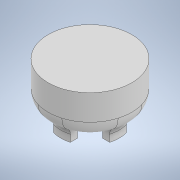
# Autodesk Inventor part: lower joint
Saved by Autodesk Inventor 2022 (Build 260153000, 153)
## iProperties
Created: 2022-03-14
Part Number: lower joint
Material: Generic
Document SubType Name: Modeling
Designer: RNG3nius
Density: 1 g/cm^3
Appearance: Default
Author: RNG3nius
Autodesk Inventor part; units mm, degrees
ref_plane "YZ Plane" through (0, 0, 0) normal (1, 0, 0) x (0, 1, 0)
ref_plane "XZ Plane" through (0, 0, 0) normal (0, 1, 0) x (-1, 0, 0)
ref_plane "XY Plane" through (0, 0, 0) normal (0, 0, 1) x (1, 0, 0)
sketch "Sketch1" plane through (0, 0, 0) normal (0, 1, 0) x (-1, 0, 0)
  circle A0 centre (0, 0) radius 5
  dimension "d0" = 10
  constraints: 1 centre point, 1 coincident
  measures "d0" diameter of A0
extrude "Extrusion1" add sketch "Sketch1" along normal blind 5
sketch "Sketch2" plane through (0, 0, 0) normal (0, -1, 0) x (1, 0, 0)
  circle A0 centre (0, 0) radius 3.5
  line L0 (1, -2.5) -> (-1, -2.5)
  line L1 (-1, -2.5) -> (-1, -4.5)
  line L2 (-1, -4.5) -> (1, -4.5)
  line L3 (1, -4.5) -> (1, -2.5)
  line L4 (1, -2.5) -> (-1, -4.5) construction
  line L5 (-1, -2.5) -> (1, -4.5) construction
  line L6 (4.5, 1) -> (2.5, 1)
  line L7 (2.5, 1) -> (2.5, -1)
  line L8 (2.5, -1) -> (4.5, -1)
  line L9 (4.5, -1) -> (4.5, 1)
  line L10 (4.5, 1) -> (2.5, -1) construction
  line L11 (2.5, 1) -> (4.5, -1) construction
  line L12 (1, 4.5) -> (-1, 4.5)
  line L13 (-1, 4.5) -> (-1, 2.5)
  line L14 (-1, 2.5) -> (1, 2.5)
  line L15 (1, 2.5) -> (1, 4.5)
  line L16 (1, 4.5) -> (-1, 2.5) construction
  line L17 (-1, 4.5) -> (1, 2.5) construction
  line L18 (-4.5, 1) -> (-2.5, 1)
  line L19 (-2.5, 1) -> (-2.5, -1)
  line L20 (-2.5, -1) -> (-4.5, -1)
  line L21 (-4.5, -1) -> (-4.5, 1)
  line L22 (-4.5, 1) -> (-2.5, -1) construction
  line L23 (-2.5, 1) -> (-4.5, -1) construction
  point P0 (0, -3.5)
  point P1 (3.5, 0)
  point P2 (0, 3.5)
  point P3 (-3.5, 0)
  point P4 (-3.3541, 1)
  point P5 (-3.3541, -1)
  point P6 (-1, -3.3541)
  point P7 (1, -3.3541)
  point P8 (3.3541, -1)
  point P9 (3.3541, 1)
  point P10 (1, 3.3541)
  point P11 (-1, 3.3541)
  dimension "d3" = 7
  dimension "d4" = 2
  dimension "d5" = 2
  dimension "d6" = 2
  dimension "d7" = 2
  dimension "d8" = 2
  dimension "d9" = 2
  dimension "d10" = 2
  dimension "d11" = 2
  constraints: 48 end point, 8 midpoint, 8 parallel, 4 horizontal, 4 perpendicular, 4 point on circle, 2 point on line, 1 centre point, 1 coincident
  measures "d3" diameter of A0
  measures "d4" distance of L2.end L1.end
  measures "d5" distance of L1.end L0.end
  measures "d6" distance of L8.end L7.end
  measures "d7" distance of L7.end L6.end
  measures "d8" distance of L14.end L13.end
  measures "d9" distance of L13.end L12.end
  measures "d10" distance of L19.end L20.end
  measures "d11" distance of L18.end L19.end
sketch "Sketch3" plane through (0, 0, 0) normal (0, -1, 0) x (1, 0, 0)
  circle A0 centre (0, 0) radius 3.5
  constraints: 1 centre point, 1 coincident
extrude "Extrusion3" cut sketch "Sketch3" against normal blind 1
extrude "Extrusion4" add sketch "Sketch2" along normal mid plane 3 contours A0 L8 L7 L6 | L15 L14 L13 A0 | A0 L1 L0 L3 | L18 L19 L20 A0
fillet "Fillet1" radius 2 1 edges at (5, 0, 0)
fillet "Fillet2" radius 1 5 edges at (0, 0, -3.5) (-3.4633, 0, 0.5053) (-3.4633, 0, -0.5053) (0, 0, 3.5) (3.5, 0, 0)
body "Solid1"
